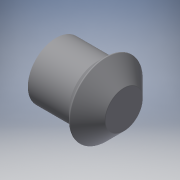
# Autodesk Inventor part: The Thing
Saved by Autodesk Inventor 2017 (Build 210142000, 142)
## iProperties
Created: 2017-03-09
Part Number: The Thing
Material: Generic
Document SubType Name: Modeling
Designer: PLTW
Density: 1 g/cm^3
Appearance: Default
Author: PLTW
Autodesk Inventor part; units mm, degrees
ref_plane "YZ Plane" through (0, 0, 0) normal (1, 0, 0) x (0, 1, 0)
ref_plane "XZ Plane" through (0, 0, 0) normal (0, 1, 0) x (-1, 0, 0)
ref_plane "XY Plane" through (0, 0, 0) normal (0, 0, 1) x (1, 0, 0)
sketch "Sketch3" plane through (0, 0, 0) normal (0, 0, 1) x (1, 0, 0)
  line L0 (-10.8841, 4.3559) -> (-10.16, 5.08)
  line L1 (-10.16, 5.08) -> (-7.62, 2.54)
  line L2 (-7.62, 2.54) -> (-7.62, -2.54)
  line L3 (-7.62, -2.54) -> (-10.16, -5.08)
  line L4 (-10.16, -5.08) -> (-10.8841, -4.3559)
  line L5 (-11.3179, 3.7425) -> (-10.16, 4.9004)
  line L6 (-10.16, 4.9004) -> (-7.747, 2.4874)
  line L7 (-7.747, 2.4874) -> (-7.747, 0)
  line L8 (-7.747, 0) -> (-16.767, 0)
  line L9 (-11.3179, 3.7425) -> (-16.767, 3.7425)
  line L10 (-16.767, 3.7425) -> (-16.767, 0)
  point P0 (0, 0)
  point P1 (-7.62, 0)
  dimension "d5" = 0.127
  dimension "d6" = 0.127
  dimension "d7" = 0.127
  constraints: 22 end point, 3 parallel, 3 perpendicular, 2 vertical, 1 horizontal, 1 horizontal alignment, 1 midpoint, 14 other
  measures "d5" distance between parallel lines of L0 L5
  measures "d6" distance between parallel lines of L1 L6
  measures "d7" distance between parallel lines of L2 L7
revolve "Revolution2" add sketch "Sketch3" angle 360 about axis through (-7.747, 0, 0) along (-1, 0, 0)
fillet "Fillet2" radius 0.127 3 edges at (-10.16, -4.9004, 0) (-11.3179, -3.7425, 0) (-7.747, -2.4874, 0)
equation "\"d6\" = d5"
equation "\"d7\" = d5"
body "Solid2"
